Autodesk Fusion 360 part; units mm, degrees
(part 2 of 4)
  line L450 (2.2628, 34.1962) -> (6.5929, 31.6962)
  line L451 (6.5929, 31.6962) -> (10.923, 34.1962)
  line L452 (10.923, 34.1962) -> (10.923, 39.1962)
  line L453 (10.923, 39.1962) -> (6.5929, 41.6962)
  line L454 (17.2532, 41.6962) -> (12.923, 39.1962)
  line L455 (12.923, 39.1962) -> (12.923, 34.1962)
  line L456 (12.923, 34.1962) -> (17.2532, 31.6962)
  line L457 (17.2532, 31.6962) -> (21.5833, 34.1962)
  line L458 (21.5833, 34.1962) -> (21.5833, 39.1962)
  line L459 (21.5833, 39.1962) -> (17.2532, 41.6962)
  line L460 (27.9134, 41.6962) -> (23.5833, 39.1962)
  line L461 (23.5833, 39.1962) -> (23.5833, 34.1962)
  line L462 (23.5833, 34.1962) -> (27.9134, 31.6962)
  line L463 (27.9134, 31.6962) -> (32.2436, 34.1962)
  line L464 (32.2436, 34.1962) -> (32.2436, 39.1962)
  line L465 (32.2436, 39.1962) -> (27.9134, 41.6962)
  line L466 (38.5737, 41.6962) -> (34.2436, 39.1962)
  line L467 (34.2436, 39.1962) -> (34.2436, 34.1962)
  line L468 (34.2436, 34.1962) -> (38.5737, 31.6962)
  line L469 (38.5737, 31.6962) -> (42.9038, 34.1962)
  line L470 (42.9038, 34.1962) -> (42.9038, 39.1962)
  line L471 (42.9038, 39.1962) -> (38.5737, 41.6962)
  line L472 (49.2339, 41.6962) -> (44.9038, 39.1962)
  line L473 (44.9038, 39.1962) -> (44.9038, 34.1962)
  line L474 (44.9038, 34.1962) -> (49.2339, 31.6962)
  line L475 (49.2339, 31.6962) -> (53.5641, 34.1962)
  line L476 (53.5641, 34.1962) -> (53.5641, 39.1962)
  line L477 (53.5641, 39.1962) -> (49.2339, 41.6962)
  line L478 (59.8942, 41.6962) -> (55.5641, 39.1962)
  line L479 (55.5641, 39.1962) -> (55.5641, 34.1962)
  line L480 (55.5641, 34.1962) -> (59.8942, 31.6962)
  line L481 (59.8942, 31.6962) -> (64.2243, 34.1962)
  line L482 (64.2243, 34.1962) -> (64.2243, 39.1962)
  line L483 (64.2243, 39.1962) -> (59.8942, 41.6962)
  line L484 (70.5544, 41.6962) -> (66.2243, 39.1962)
  line L485 (66.2243, 39.1962) -> (66.2243, 34.1962)
  line L486 (66.2243, 34.1962) -> (70.5544, 31.6962)
  line L487 (70.5544, 31.6962) -> (74.8846, 34.1962)
  line L488 (74.8846, 34.1962) -> (74.8846, 39.1962)
  line L489 (74.8846, 39.1962) -> (70.5544, 41.6962)
  line L490 (81.2147, 41.6962) -> (76.8846, 39.1962)
  line L491 (76.8846, 39.1962) -> (76.8846, 34.1962)
  line L492 (76.8846, 34.1962) -> (81.2147, 31.6962)
  line L493 (81.2147, 31.6962) -> (85.5448, 34.1962)
  line L494 (85.5448, 34.1962) -> (85.5448, 39.1962)
  line L495 (85.5448, 39.1962) -> (81.2147, 41.6962)
  line L496 (91.875, 41.6962) -> (87.5448, 39.1962)
  line L497 (87.5448, 39.1962) -> (87.5448, 34.1962)
  line L498 (87.5448, 34.1962) -> (91.875, 31.6962)
  line L499 (91.875, 31.6962) -> (96.2051, 34.1962)
  line L500 (96.2051, 34.1962) -> (96.2051, 39.1962)
  line L501 (96.2051, 39.1962) -> (91.875, 41.6962)
  line L502 (102.5352, 41.6962) -> (98.2051, 39.1962)
  line L503 (98.2051, 39.1962) -> (98.2051, 34.1962)
  line L504 (98.2051, 34.1962) -> (102.5352, 31.6962)
  line L505 (102.5352, 31.6962) -> (106.8653, 34.1962)
  line L506 (106.8653, 34.1962) -> (106.8653, 39.1962)
  line L507 (106.8653, 39.1962) -> (102.5352, 41.6962)
  line L508 (-116, 50.9282) -> (-120.3301, 48.4282)
  line L509 (-120.3301, 48.4282) -> (-120.3301, 43.4282)
  line L510 (-120.3301, 43.4282) -> (-116, 40.9282)
  line L511 (-116, 40.9282) -> (-111.6699, 43.4282)
  line L512 (-111.6699, 43.4282) -> (-111.6699, 48.4282)
  line L513 (-111.6699, 48.4282) -> (-116, 50.9282)
  line L514 (-105.3397, 50.9282) -> (-109.6699, 48.4282)
  line L515 (-109.6699, 48.4282) -> (-109.6699, 43.4282)
  line L516 (-109.6699, 43.4282) -> (-105.3397, 40.9282)
  line L517 (-105.3397, 40.9282) -> (-101.0096, 43.4282)
  line L518 (-101.0096, 43.4282) -> (-101.0096, 48.4282)
  line L519 (-101.0096, 48.4282) -> (-105.3397, 50.9282)
  line L520 (-94.6795, 50.9282) -> (-99.0096, 48.4282)
  line L521 (-99.0096, 48.4282) -> (-99.0096, 43.4282)
  line L522 (-99.0096, 43.4282) -> (-94.6795, 40.9282)
  line L523 (-94.6795, 40.9282) -> (-90.3494, 43.4282)
  line L524 (-90.3494, 43.4282) -> (-90.3494, 48.4282)
  line L525 (-90.3494, 48.4282) -> (-94.6795, 50.9282)
  line L526 (-84.0192, 50.9282) -> (-88.3494, 48.4282)
  line L527 (-88.3494, 48.4282) -> (-88.3494, 43.4282)
  line L528 (-88.3494, 43.4282) -> (-84.0192, 40.9282)
  line L529 (-84.0192, 40.9282) -> (-79.6891, 43.4282)
  line L530 (-79.6891, 43.4282) -> (-79.6891, 48.4282)
  line L531 (-79.6891, 48.4282) -> (-84.0192, 50.9282)
  line L532 (-73.359, 50.9282) -> (-77.6891, 48.4282)
  line L533 (-77.6891, 48.4282) -> (-77.6891, 43.4282)
  line L534 (-77.6891, 43.4282) -> (-73.359, 40.9282)
  line L535 (-73.359, 40.9282) -> (-69.0289, 43.4282)
  line L536 (-69.0289, 43.4282) -> (-69.0289, 48.4282)
  line L537 (-69.0289, 48.4282) -> (-73.359, 50.9282)
  line L538 (-62.6987, 50.9282) -> (-67.0289, 48.4282)
  line L539 (-67.0289, 48.4282) -> (-67.0289, 43.4282)
  line L540 (-67.0289, 43.4282) -> (-62.6987, 40.9282)
  line L541 (-62.6987, 40.9282) -> (-58.3686, 43.4282)
  line L542 (-58.3686, 43.4282) -> (-58.3686, 48.4282)
  line L543 (-58.3686, 48.4282) -> (-62.6987, 50.9282)
  line L544 (-52.0385, 50.9282) -> (-56.3686, 48.4282)
  line L545 (-56.3686, 48.4282) -> (-56.3686, 43.4282)
  line L546 (-56.3686, 43.4282) -> (-52.0385, 40.9282)
  line L547 (-52.0385, 40.9282) -> (-47.7083, 43.4282)
  line L548 (-47.7083, 43.4282) -> (-47.7083, 48.4282)
  line L549 (-47.7083, 48.4282) -> (-52.0385, 50.9282)
  line L550 (-41.3782, 50.9282) -> (-45.7083, 48.4282)
  line L551 (-45.7083, 48.4282) -> (-45.7083, 43.4282)
  line L552 (-45.7083, 43.4282) -> (-41.3782, 40.9282)
  line L553 (-41.3782, 40.9282) -> (-37.0481, 43.4282)
  line L554 (-37.0481, 43.4282) -> (-37.0481, 48.4282)
  line L555 (-37.0481, 48.4282) -> (-41.3782, 50.9282)
  line L556 (-30.718, 50.9282) -> (-35.0481, 48.4282)
  line L557 (-35.0481, 48.4282) -> (-35.0481, 43.4282)
  line L558 (-35.0481, 43.4282) -> (-30.718, 40.9282)
  line L559 (-30.718, 40.9282) -> (-26.3878, 43.4282)
  line L560 (-26.3878, 43.4282) -> (-26.3878, 48.4282)
  line L561 (-26.3878, 48.4282) -> (-30.718, 50.9282)
  line L562 (-20.0577, 50.9282) -> (-24.3878, 48.4282)
  line L563 (-24.3878, 48.4282) -> (-24.3878, 43.4282)
  line L564 (-24.3878, 43.4282) -> (-20.0577, 40.9282)
  line L565 (-20.0577, 40.9282) -> (-15.7276, 43.4282)
  line L566 (-15.7276, 43.4282) -> (-15.7276, 48.4282)
  line L567 (-15.7276, 48.4282) -> (-20.0577, 50.9282)
  line L568 (-9.3975, 50.9282) -> (-13.7276, 48.4282)
  line L569 (-13.7276, 48.4282) -> (-13.7276, 43.4282)
  line L570 (-13.7276, 43.4282) -> (-9.3975, 40.9282)
  line L571 (-9.3975, 40.9282) -> (-5.0673, 43.4282)
  line L572 (-5.0673, 43.4282) -> (-5.0673, 48.4282)
  line L573 (-5.0673, 48.4282) -> (-9.3975, 50.9282)
  line L574 (1.2628, 50.9282) -> (-3.0673, 48.4282)
  line L575 (-3.0673, 48.4282) -> (-3.0673, 43.4282)
  line L576 (-3.0673, 43.4282) -> (1.2628, 40.9282)
  line L577 (1.2628, 40.9282) -> (5.5929, 43.4282)
  line L578 (5.5929, 43.4282) -> (5.5929, 48.4282)
  line L579 (5.5929, 48.4282) -> (1.2628, 50.9282)
  line L580 (11.923, 50.9282) -> (7.5929, 48.4282)
  line L581 (7.5929, 48.4282) -> (7.5929, 43.4282)
  line L582 (7.5929, 43.4282) -> (11.923, 40.9282)
  line L583 (11.923, 40.9282) -> (16.2532, 43.4282)
  line L584 (16.2532, 43.4282) -> (16.2532, 48.4282)
  line L585 (16.2532, 48.4282) -> (11.923, 50.9282)
  line L586 (22.5833, 50.9282) -> (18.2532, 48.4282)
  line L587 (18.2532, 48.4282) -> (18.2532, 43.4282)
  line L588 (18.2532, 43.4282) -> (22.5833, 40.9282)
  line L589 (22.5833, 40.9282) -> (26.9134, 43.4282)
  line L590 (26.9134, 43.4282) -> (26.9134, 48.4282)
  line L591 (26.9134, 48.4282) -> (22.5833, 50.9282)
  line L592 (33.2436, 50.9282) -> (28.9134, 48.4282)
  line L593 (28.9134, 48.4282) -> (28.9134, 43.4282)
  line L594 (28.9134, 43.4282) -> (33.2436, 40.9282)
  line L595 (33.2436, 40.9282) -> (37.5737, 43.4282)
  line L596 (37.5737, 43.4282) -> (37.5737, 48.4282)
  line L597 (37.5737, 48.4282) -> (33.2436, 50.9282)
  line L598 (43.9038, 50.9282) -> (39.5737, 48.4282)
  line L599 (39.5737, 48.4282) -> (39.5737, 43.4282)
  line L600 (39.5737, 43.4282) -> (43.9038, 40.9282)
  line L601 (43.9038, 40.9282) -> (48.2339, 43.4282)
  line L602 (48.2339, 43.4282) -> (48.2339, 48.4282)
  line L603 (48.2339, 48.4282) -> (43.9038, 50.9282)
  line L604 (54.5641, 50.9282) -> (50.2339, 48.4282)
  line L605 (50.2339, 48.4282) -> (50.2339, 43.4282)
  line L606 (50.2339, 43.4282) -> (54.5641, 40.9282)
  line L607 (54.5641, 40.9282) -> (58.8942, 43.4282)
  line L608 (58.8942, 43.4282) -> (58.8942, 48.4282)
  line L609 (58.8942, 48.4282) -> (54.5641, 50.9282)
  line L610 (65.2243, 50.9282) -> (60.8942, 48.4282)
  line L611 (60.8942, 48.4282) -> (60.8942, 43.4282)
  line L612 (60.8942, 43.4282) -> (65.2243, 40.9282)
  line L613 (65.2243, 40.9282) -> (69.5544, 43.4282)
  line L614 (69.5544, 43.4282) -> (69.5544, 48.4282)
  line L615 (69.5544, 48.4282) -> (65.2243, 50.9282)
  line L616 (75.8846, 50.9282) -> (71.5544, 48.4282)
  line L617 (71.5544, 48.4282) -> (71.5544, 43.4282)
  line L618 (71.5544, 43.4282) -> (75.8846, 40.9282)
  line L619 (75.8846, 40.9282) -> (80.2147, 43.4282)
  line L620 (80.2147, 43.4282) -> (80.2147, 48.4282)
  line L621 (80.2147, 48.4282) -> (75.8846, 50.9282)
  line L622 (86.5448, 50.9282) -> (82.2147, 48.4282)
  line L623 (82.2147, 48.4282) -> (82.2147, 43.4282)
  line L624 (82.2147, 43.4282) -> (86.5448, 40.9282)
  line L625 (86.5448, 40.9282) -> (90.875, 43.4282)
  line L626 (90.875, 43.4282) -> (90.875, 48.4282)
  line L627 (90.875, 48.4282) -> (86.5448, 50.9282)
  line L628 (97.2051, 50.9282) -> (92.875, 48.4282)
  line L629 (92.875, 48.4282) -> (92.875, 43.4282)
  line L630 (92.875, 43.4282) -> (97.2051, 40.9282)
  line L631 (97.2051, 40.9282) -> (101.5352, 43.4282)
  line L632 (101.5352, 43.4282) -> (101.5352, 48.4282)
  line L633 (101.5352, 48.4282) -> (97.2051, 50.9282)
  line L634 (-110.6699, 60.1603) -> (-115, 57.6603)
  line L635 (-115, 57.6603) -> (-115, 52.6603)
  line L636 (-115, 52.6603) -> (-110.6699, 50.1603)
  line L637 (-110.6699, 50.1603) -> (-106.3397, 52.6603)
  line L638 (-106.3397, 52.6603) -> (-106.3397, 57.6603)
  line L639 (-106.3397, 57.6603) -> (-110.6699, 60.1603)
  line L640 (-100.0096, 60.1603) -> (-104.3397, 57.6603)
  line L641 (-104.3397, 57.6603) -> (-104.3397, 52.6603)
  line L642 (-104.3397, 52.6603) -> (-100.0096, 50.1603)
  line L643 (-100.0096, 50.1603) -> (-95.6795, 52.6603)
  line L644 (-95.6795, 52.6603) -> (-95.6795, 57.6603)
  line L645 (-95.6795, 57.6603) -> (-100.0096, 60.1603)
  line L646 (-89.3494, 60.1603) -> (-93.6795, 57.6603)
  line L647 (-93.6795, 57.6603) -> (-93.6795, 52.6603)
  line L648 (-93.6795, 52.6603) -> (-89.3494, 50.1603)
  line L649 (-89.3494, 50.1603) -> (-85.0192, 52.6603)
  line L650 (-85.0192, 52.6603) -> (-85.0192, 57.6603)
  line L651 (-85.0192, 57.6603) -> (-89.3494, 60.1603)
  line L652 (-78.6891, 60.1603) -> (-83.0192, 57.6603)
  line L653 (-83.0192, 57.6603) -> (-83.0192, 52.6603)
  line L654 (-83.0192, 52.6603) -> (-78.6891, 50.1603)
  line L655 (-78.6891, 50.1603) -> (-74.359, 52.6603)
  line L656 (-74.359, 52.6603) -> (-74.359, 57.6603)
  line L657 (-74.359, 57.6603) -> (-78.6891, 60.1603)
  line L658 (-68.0289, 60.1603) -> (-72.359, 57.6603)
  line L659 (-72.359, 57.6603) -> (-72.359, 52.6603)
  line L660 (-72.359, 52.6603) -> (-68.0289, 50.1603)
  line L661 (-68.0289, 50.1603) -> (-63.6987, 52.6603)
  line L662 (-63.6987, 52.6603) -> (-63.6987, 57.6603)
  line L663 (-63.6987, 57.6603) -> (-68.0289, 60.1603)
  line L664 (-57.3686, 60.1603) -> (-61.6987, 57.6603)
  line L665 (-61.6987, 57.6603) -> (-61.6987, 52.6603)
  line L666 (-61.6987, 52.6603) -> (-57.3686, 50.1603)
  line L667 (-57.3686, 50.1603) -> (-53.0385, 52.6603)
  line L668 (-53.0385, 52.6603) -> (-53.0385, 57.6603)
  line L669 (-53.0385, 57.6603) -> (-57.3686, 60.1603)
  line L670 (-46.7083, 60.1603) -> (-51.0385, 57.6603)
  line L671 (-51.0385, 57.6603) -> (-51.0385, 52.6603)
  line L672 (-51.0385, 52.6603) -> (-46.7083, 50.1603)
  line L673 (-46.7083, 50.1603) -> (-42.3782, 52.6603)
  line L674 (-42.3782, 52.6603) -> (-42.3782, 57.6603)
  line L675 (-42.3782, 57.6603) -> (-46.7083, 60.1603)
  line L676 (-36.0481, 60.1603) -> (-40.3782, 57.6603)
  line L677 (-40.3782, 57.6603) -> (-40.3782, 52.6603)
  line L678 (-40.3782, 52.6603) -> (-36.0481, 50.1603)
  line L679 (-36.0481, 50.1603) -> (-31.718, 52.6603)
  line L680 (-31.718, 52.6603) -> (-31.718, 57.6603)
  line L681 (-31.718, 57.6603) -> (-36.0481, 60.1603)
  line L682 (-25.3878, 60.1603) -> (-29.718, 57.6603)
  line L683 (-29.718, 57.6603) -> (-29.718, 52.6603)
  line L684 (-29.718, 52.6603) -> (-25.3878, 50.1603)
  line L685 (-25.3878, 50.1603) -> (-21.0577, 52.6603)
  line L686 (-21.0577, 52.6603) -> (-21.0577, 57.6603)
  line L687 (-21.0577, 57.6603) -> (-25.3878, 60.1603)
  line L688 (-14.7276, 60.1603) -> (-19.0577, 57.6603)
  line L689 (-19.0577, 57.6603) -> (-19.0577, 52.6603)
  line L690 (-19.0577, 52.6603) -> (-14.7276, 50.1603)
  line L691 (-14.7276, 50.1603) -> (-10.3975, 52.6603)
  line L692 (-10.3975, 52.6603) -> (-10.3975, 57.6603)
  line L693 (-10.3975, 57.6603) -> (-14.7276, 60.1603)
  line L694 (-4.0673, 60.1603) -> (-8.3975, 57.6603)
  line L695 (-8.3975, 57.6603) -> (-8.3975, 52.6603)
  line L696 (-8.3975, 52.6603) -> (-4.0673, 50.1603)
  line L697 (-4.0673, 50.1603) -> (0.2628, 52.6603)
  line L698 (0.2628, 52.6603) -> (0.2628, 57.6603)
  line L699 (0.2628, 57.6603) -> (-4.0673, 60.1603)
  line L700 (6.5929, 60.1603) -> (2.2628, 57.6603)
  line L701 (2.2628, 57.6603) -> (2.2628, 52.6603)
  line L702 (2.2628, 52.6603) -> (6.5929, 50.1603)
  line L703 (6.5929, 50.1603) -> (10.923, 52.6603)
  line L704 (10.923, 52.6603) -> (10.923, 57.6603)
  line L705 (10.923, 57.6603) -> (6.5929, 60.1603)
  line L706 (17.2532, 60.1603) -> (12.923, 57.6603)
  line L707 (12.923, 57.6603) -> (12.923, 52.6603)
  line L708 (12.923, 52.6603) -> (17.2532, 50.1603)
  line L709 (17.2532, 50.1603) -> (21.5833, 52.6603)
  line L710 (21.5833, 52.6603) -> (21.5833, 57.6603)
  line L711 (21.5833, 57.6603) -> (17.2532, 60.1603)
  line L712 (27.9134, 60.1603) -> (23.5833, 57.6603)
  line L713 (23.5833, 57.6603) -> (23.5833, 52.6603)
  line L714 (23.5833, 52.6603) -> (27.9134, 50.1603)
  line L715 (27.9134, 50.1603) -> (32.2436, 52.6603)
  line L716 (32.2436, 52.6603) -> (32.2436, 57.6603)
  line L717 (32.2436, 57.6603) -> (27.9134, 60.1603)
  line L718 (38.5737, 60.1603) -> (34.2436, 57.6603)
  line L719 (34.2436, 57.6603) -> (34.2436, 52.6603)
  line L720 (34.2436, 52.6603) -> (38.5737, 50.1603)
  line L721 (38.5737, 50.1603) -> (42.9038, 52.6603)
  line L722 (42.9038, 52.6603) -> (42.9038, 57.6603)
  line L723 (42.9038, 57.6603) -> (38.5737, 60.1603)
  line L724 (49.2339, 60.1603) -> (44.9038, 57.6603)
  line L725 (44.9038, 57.6603) -> (44.9038, 52.6603)
  line L726 (44.9038, 52.6603) -> (49.2339, 50.1603)
  line L727 (49.2339, 50.1603) -> (53.5641, 52.6603)
  line L728 (53.5641, 52.6603) -> (53.5641, 57.6603)
  line L729 (53.5641, 57.6603) -> (49.2339, 60.1603)
  line L730 (59.8942, 60.1603) -> (55.5641, 57.6603)
  line L731 (55.5641, 57.6603) -> (55.5641, 52.6603)
  line L732 (55.5641, 52.6603) -> (59.8942, 50.1603)
  line L733 (59.8942, 50.1603) -> (64.2243, 52.6603)
  line L734 (64.2243, 52.6603) -> (64.2243, 57.6603)
  line L735 (64.2243, 57.6603) -> (59.8942, 60.1603)
  line L736 (70.5544, 60.1603) -> (66.2243, 57.6603)
  line L737 (66.2243, 57.6603) -> (66.2243, 52.6603)
  line L738 (66.2243, 52.6603) -> (70.5544, 50.1603)
  line L739 (70.5544, 50.1603) -> (74.8846, 52.6603)
  line L740 (74.8846, 52.6603) -> (74.8846, 57.6603)
  line L741 (74.8846, 57.6603) -> (70.5544, 60.1603)
  line L742 (81.2147, 60.1603) -> (76.8846, 57.6603)
  line L743 (76.8846, 57.6603) -> (76.8846, 52.6603)
  line L744 (76.8846, 52.6603) -> (81.2147, 50.1603)
  line L745 (81.2147, 50.1603) -> (85.5448, 52.6603)
  line L746 (85.5448, 52.6603) -> (85.5448, 57.6603)
  line L747 (85.5448, 57.6603) -> (81.2147, 60.1603)
  line L748 (91.875, 60.1603) -> (87.5448, 57.6603)
  line L749 (87.5448, 57.6603) -> (87.5448, 52.6603)
  line L750 (87.5448, 52.6603) -> (91.875, 50.1603)
  line L751 (91.875, 50.1603) -> (96.2051, 52.6603)
  line L752 (96.2051, 52.6603) -> (96.2051, 57.6603)
  line L753 (96.2051, 57.6603) -> (91.875, 60.1603)
  line L754 (102.5352, 60.1603) -> (98.2051, 57.6603)
  line L755 (98.2051, 57.6603) -> (98.2051, 52.6603)
  line L756 (98.2051, 52.6603) -> (102.5352, 50.1603)
  line L757 (102.5352, 50.1603) -> (106.8653, 52.6603)
  line L758 (106.8653, 52.6603) -> (106.8653, 57.6603)
  line L759 (106.8653, 57.6603) -> (102.5352, 60.1603)
  line L760 (-116, 69.3923) -> (-120.3301, 66.8923)
  line L761 (-120.3301, 66.8923) -> (-120.3301, 61.8923)
  line L762 (-120.3301, 61.8923) -> (-116, 59.3923)
  line L763 (-116, 59.3923) -> (-111.6699, 61.8923)
  line L764 (-111.6699, 61.8923) -> (-111.6699, 66.8923)
  line L765 (-111.6699, 66.8923) -> (-116, 69.3923)
  line L766 (-105.3397, 69.3923) -> (-109.6699, 66.8923)
  line L767 (-109.6699, 66.8923) -> (-109.6699, 61.8923)
  line L768 (-109.6699, 61.8923) -> (-105.3397, 59.3923)
  line L769 (-105.3397, 59.3923) -> (-101.0096, 61.8923)
  line L770 (-101.0096, 61.8923) -> (-101.0096, 66.8923)
  line L771 (-101.0096, 66.8923) -> (-105.3397, 69.3923)
  line L772 (-94.6795, 69.3923) -> (-99.0096, 66.8923)
  line L773 (-99.0096, 66.8923) -> (-99.0096, 61.8923)
  line L774 (-99.0096, 61.8923) -> (-94.6795, 59.3923)
  line L775 (-94.6795, 59.3923) -> (-90.3494, 61.8923)
  line L776 (-90.3494, 61.8923) -> (-90.3494, 66.8923)
  line L777 (-90.3494, 66.8923) -> (-94.6795, 69.3923)
  line L778 (-84.0192, 69.3923) -> (-88.3494, 66.8923)
  line L779 (-88.3494, 66.8923) -> (-88.3494, 61.8923)
  line L780 (-88.3494, 61.8923) -> (-84.0192, 59.3923)
  line L781 (-84.0192, 59.3923) -> (-79.6891, 61.8923)
  line L782 (-79.6891, 61.8923) -> (-79.6891, 66.8923)
  line L783 (-79.6891, 66.8923) -> (-84.0192, 69.3923)
  line L784 (-73.359, 69.3923) -> (-77.6891, 66.8923)
  line L785 (-77.6891, 66.8923) -> (-77.6891, 61.8923)
  line L786 (-77.6891, 61.8923) -> (-73.359, 59.3923)
  line L787 (-73.359, 59.3923) -> (-69.0289, 61.8923)
  line L788 (-69.0289, 61.8923) -> (-69.0289, 66.8923)
  line L789 (-69.0289, 66.8923) -> (-73.359, 69.3923)
  line L790 (-62.6987, 69.3923) -> (-67.0289, 66.8923)
  line L791 (-67.0289, 66.8923) -> (-67.0289, 61.8923)
  line L792 (-67.0289, 61.8923) -> (-62.6987, 59.3923)
  line L793 (-62.6987, 59.3923) -> (-58.3686, 61.8923)
  line L794 (-58.3686, 61.8923) -> (-58.3686, 66.8923)
  line L795 (-58.3686, 66.8923) -> (-62.6987, 69.3923)
  line L796 (-52.0385, 69.3923) -> (-56.3686, 66.8923)
  line L797 (-56.3686, 66.8923) -> (-56.3686, 61.8923)
  line L798 (-56.3686, 61.8923) -> (-52.0385, 59.3923)
  line L799 (-52.0385, 59.3923) -> (-47.7083, 61.8923)
  line L800 (-47.7083, 61.8923) -> (-47.7083, 66.8923)
  line L801 (-47.7083, 66.8923) -> (-52.0385, 69.3923)
  line L802 (-41.3782, 69.3923) -> (-45.7083, 66.8923)
  line L803 (-45.7083, 66.8923) -> (-45.7083, 61.8923)
  line L804 (-45.7083, 61.8923) -> (-41.3782, 59.3923)
  line L805 (-41.3782, 59.3923) -> (-37.0481, 61.8923)
  line L806 (-37.0481, 61.8923) -> (-37.0481, 66.8923)
  line L807 (-37.0481, 66.8923) -> (-41.3782, 69.3923)
  line L808 (-30.718, 69.3923) -> (-35.0481, 66.8923)
  line L809 (-35.0481, 66.8923) -> (-35.0481, 61.8923)
  line L810 (-35.0481, 61.8923) -> (-30.718, 59.3923)
  line L811 (-30.718, 59.3923) -> (-26.3878, 61.8923)
  line L812 (-26.3878, 61.8923) -> (-26.3878, 66.8923)
  line L813 (-26.3878, 66.8923) -> (-30.718, 69.3923)
  line L814 (-20.0577, 69.3923) -> (-24.3878, 66.8923)
  line L815 (-24.3878, 66.8923) -> (-24.3878, 61.8923)
  line L816 (-24.3878, 61.8923) -> (-20.0577, 59.3923)
  line L817 (-20.0577, 59.3923) -> (-15.7276, 61.8923)
  line L818 (-15.7276, 61.8923) -> (-15.7276, 66.8923)
  line L819 (-15.7276, 66.8923) -> (-20.0577, 69.3923)
  line L820 (-9.3975, 69.3923) -> (-13.7276, 66.8923)
  line L821 (-13.7276, 66.8923) -> (-13.7276, 61.8923)
  line L822 (-13.7276, 61.8923) -> (-9.3975, 59.3923)
  line L823 (-9.3975, 59.3923) -> (-5.0673, 61.8923)
  line L824 (-5.0673, 61.8923) -> (-5.0673, 66.8923)
  line L825 (-5.0673, 66.8923) -> (-9.3975, 69.3923)
  line L826 (1.2628, 69.3923) -> (-3.0673, 66.8923)
  line L827 (-3.0673, 66.8923) -> (-3.0673, 61.8923)
  line L828 (-3.0673, 61.8923) -> (1.2628, 59.3923)
  line L829 (1.2628, 59.3923) -> (5.5929, 61.8923)
  line L830 (5.5929, 61.8923) -> (5.5929, 66.8923)
  line L831 (5.5929, 66.8923) -> (1.2628, 69.3923)
  line L832 (11.923, 69.3923) -> (7.5929, 66.8923)
  line L833 (7.5929, 66.8923) -> (7.5929, 61.8923)
  line L834 (7.5929, 61.8923) -> (11.923, 59.3923)
  line L835 (11.923, 59.3923) -> (16.2532, 61.8923)
  line L836 (16.2532, 61.8923) -> (16.2532, 66.8923)
  line L837 (16.2532, 66.8923) -> (11.923, 69.3923)
  line L838 (22.5833, 69.3923) -> (18.2532, 66.8923)
  line L839 (18.2532, 66.8923) -> (18.2532, 61.8923)
  line L840 (18.2532, 61.8923) -> (22.5833, 59.3923)
  line L841 (22.5833, 59.3923) -> (26.9134, 61.8923)
  line L842 (26.9134, 61.8923) -> (26.9134, 66.8923)
  line L843 (26.9134, 66.8923) -> (22.5833, 69.3923)
  line L844 (33.2436, 69.3923) -> (28.9134, 66.8923)
  line L845 (28.9134, 66.8923) -> (28.9134, 61.8923)
  line L846 (28.9134, 61.8923) -> (33.2436, 59.3923)
  line L847 (33.2436, 59.3923) -> (37.5737, 61.8923)
  line L848 (37.5737, 61.8923) -> (37.5737, 66.8923)
  line L849 (37.5737, 66.8923) -> (33.2436, 69.3923)
  line L850 (43.9038, 69.3923) -> (39.5737, 66.8923)
  line L851 (39.5737, 66.8923) -> (39.5737, 61.8923)
  line L852 (39.5737, 61.8923) -> (43.9038, 59.3923)
  line L853 (43.9038, 59.3923) -> (48.2339, 61.8923)
  line L854 (48.2339, 61.8923) -> (48.2339, 66.8923)
  line L855 (48.2339, 66.8923) -> (43.9038, 69.3923)
  line L856 (54.5641, 69.3923) -> (50.2339, 66.8923)
  line L857 (50.2339, 66.8923) -> (50.2339, 61.8923)
  line L858 (50.2339, 61.8923) -> (54.5641, 59.3923)
  line L859 (54.5641, 59.3923) -> (58.8942, 61.8923)
  line L860 (58.8942, 61.8923) -> (58.8942, 66.8923)
  line L861 (58.8942, 66.8923) -> (54.5641, 69.3923)
  line L862 (65.2243, 69.3923) -> (60.8942, 66.8923)
  line L863 (60.8942, 66.8923) -> (60.8942, 61.8923)
  line L864 (60.8942, 61.8923) -> (65.2243, 59.3923)
  line L865 (65.2243, 59.3923) -> (69.5544, 61.8923)
  line L866 (69.5544, 61.8923) -> (69.5544, 66.8923)
  line L867 (69.5544, 66.8923) -> (65.2243, 69.3923)
  line L868 (75.8846, 69.3923) -> (71.5544, 66.8923)
  line L869 (71.5544, 66.8923) -> (71.5544, 61.8923)
  line L870 (71.5544, 61.8923) -> (75.8846, 59.3923)
  line L871 (75.8846, 59.3923) -> (80.2147, 61.8923)
  line L872 (80.2147, 61.8923) -> (80.2147, 66.8923)
  line L873 (80.2147, 66.8923) -> (75.8846, 69.3923)
  line L874 (86.5448, 69.3923) -> (82.2147, 66.8923)
  line L875 (82.2147, 66.8923) -> (82.2147, 61.8923)
  line L876 (82.2147, 61.8923) -> (86.5448, 59.3923)
  line L877 (86.5448, 59.3923) -> (90.875, 61.8923)
  line L878 (90.875, 61.8923) -> (90.875, 66.8923)
  line L879 (90.875, 66.8923) -> (86.5448, 69.3923)
  line L880 (97.2051, 69.3923) -> (92.875, 66.8923)
  line L881 (92.875, 66.8923) -> (92.875, 61.8923)
  line L882 (92.875, 61.8923) -> (97.2051, 59.3923)
  line L883 (97.2051, 59.3923) -> (101.5352, 61.8923)
  line L884 (101.5352, 61.8923) -> (101.5352, 66.8923)
  line L885 (101.5352, 66.8923) -> (97.2051, 69.3923)
  line L886 (-110.6699, 78.6244) -> (-115, 76.1244)
  line L887 (-115, 76.1244) -> (-115, 71.1244)
  line L888 (-115, 71.1244) -> (-110.6699, 68.6244)
  line L889 (-110.6699, 68.6244) -> (-106.3397, 71.1244)
  line L890 (-106.3397, 71.1244) -> (-106.3397, 76.1244)
  line L891 (-106.3397, 76.1244) -> (-110.6699, 78.6244)
  line L892 (-100.0096, 78.6244) -> (-104.3397, 76.1244)
  line L893 (-104.3397, 76.1244) -> (-104.3397, 71.1244)
  line L894 (-104.3397, 71.1244) -> (-100.0096, 68.6244)
  line L895 (-100.0096, 68.6244) -> (-95.6795, 71.1244)
  line L896 (-95.6795, 71.1244) -> (-95.6795, 76.1244)
  line L897 (-95.6795, 76.1244) -> (-100.0096, 78.6244)
  line L898 (-89.3494, 78.6244) -> (-93.6795, 76.1244)
  line L899 (-93.6795, 76.1244) -> (-93.6795, 71.1244)
  line L900 (-93.6795, 71.1244) -> (-89.3494, 68.6244)
  line L901 (-89.3494, 68.6244) -> (-85.0192, 71.1244)
  line L902 (-85.0192, 71.1244) -> (-85.0192, 76.1244)
  line L903 (-85.0192, 76.1244) -> (-89.3494, 78.6244)
  line L904 (-78.6891, 78.6244) -> (-83.0192, 76.1244)
  line L905 (-83.0192, 76.1244) -> (-83.0192, 71.1244)
  line L906 (-83.0192, 71.1244) -> (-78.6891, 68.6244)
  line L907 (-78.6891, 68.6244) -> (-74.359, 71.1244)
  line L908 (-74.359, 71.1244) -> (-74.359, 76.1244)
  line L909 (-74.359, 76.1244) -> (-78.6891, 78.6244)
  line L910 (-68.0289, 78.6244) -> (-72.359, 76.1244)
  line L911 (-72.359, 76.1244) -> (-72.359, 71.1244)
  line L912 (-72.359, 71.1244) -> (-68.0289, 68.6244)
  line L913 (-68.0289, 68.6244) -> (-63.6987, 71.1244)
  line L914 (-63.6987, 71.1244) -> (-63.6987, 76.1244)
  line L915 (-63.6987, 76.1244) -> (-68.0289, 78.6244)
  line L916 (-57.3686, 78.6244) -> (-61.6987, 76.1244)
  line L917 (-61.6987, 76.1244) -> (-61.6987, 71.1244)
  line L918 (-61.6987, 71.1244) -> (-57.3686, 68.6244)
  line L919 (-57.3686, 68.6244) -> (-53.0385, 71.1244)
  line L920 (-53.0385, 71.1244) -> (-53.0385, 76.1244)
  line L921 (-53.0385, 76.1244) -> (-57.3686, 78.6244)
  line L922 (-46.7083, 78.6244) -> (-51.0385, 76.1244)
  line L923 (-51.0385, 76.1244) -> (-51.0385, 71.1244)
  line L924 (-51.0385, 71.1244) -> (-46.7083, 68.6244)
  line L925 (-46.7083, 68.6244) -> (-42.3782, 71.1244)
  line L926 (-42.3782, 71.1244) -> (-42.3782, 76.1244)
  line L927 (-42.3782, 76.1244) -> (-46.7083, 78.6244)
  line L928 (-36.0481, 78.6244) -> (-40.3782, 76.1244)
  line L929 (-40.3782, 76.1244) -> (-40.3782, 71.1244)
  line L930 (-40.3782, 71.1244) -> (-36.0481, 68.6244)
  line L931 (-36.0481, 68.6244) -> (-31.718, 71.1244)
  line L932 (-31.718, 71.1244) -> (-31.718, 76.1244)
  line L933 (-31.718, 76.1244) -> (-36.0481, 78.6244)
  line L934 (-25.3878, 78.6244) -> (-29.718, 76.1244)
  line L935 (-29.718, 76.1244) -> (-29.718, 71.1244)
  line L936 (-29.718, 71.1244) -> (-25.3878, 68.6244)
  line L937 (-25.3878, 68.6244) -> (-21.0577, 71.1244)
  line L938 (-21.0577, 71.1244) -> (-21.0577, 76.1244)
  line L939 (-21.0577, 76.1244) -> (-25.3878, 78.6244)
  line L940 (-14.7276, 78.6244) -> (-19.0577, 76.1244)
  line L941 (-19.0577, 76.1244) -> (-19.0577, 71.1244)
  line L942 (-19.0577, 71.1244) -> (-14.7276, 68.6244)
  line L943 (-14.7276, 68.6244) -> (-10.3975, 71.1244)
  line L944 (-10.3975, 71.1244) -> (-10.3975, 76.1244)
  line L945 (-10.3975, 76.1244) -> (-14.7276, 78.6244)
  line L946 (-4.0673, 78.6244) -> (-8.3975, 76.1244)
  line L947 (-8.3975, 76.1244) -> (-8.3975, 71.1244)
  line L948 (-8.3975, 71.1244) -> (-4.0673, 68.6244)
  line L949 (-4.0673, 68.6244) -> (0.2628, 71.1244)
  line L950 (0.2628, 71.1244) -> (0.2628, 76.1244)
  line L951 (0.2628, 76.1244) -> (-4.0673, 78.6244)
  line L952 (6.5929, 78.6244) -> (2.2628, 76.1244)
  line L953 (2.2628, 76.1244) -> (2.2628, 71.1244)
  line L954 (2.2628, 71.1244) -> (6.5929, 68.6244)
  line L955 (6.5929, 68.6244) -> (10.923, 71.1244)
  line L956 (10.923, 71.1244) -> (10.923, 76.1244)
  line L957 (10.923, 76.1244) -> (6.5929, 78.6244)
  line L958 (17.2532, 78.6244) -> (12.923, 76.1244)
  line L959 (12.923, 76.1244) -> (12.923, 71.1244)
  line L960 (12.923, 71.1244) -> (17.2532, 68.6244)
  line L961 (17.2532, 68.6244) -> (21.5833, 71.1244)
  line L962 (21.5833, 71.1244) -> (21.5833, 76.1244)
  line L963 (21.5833, 76.1244) -> (17.2532, 78.6244)
  line L964 (27.9134, 78.6244) -> (23.5833, 76.1244)
  line L965 (23.5833, 76.1244) -> (23.5833, 71.1244)
  line L966 (23.5833, 71.1244) -> (27.9134, 68.6244)
  line L967 (27.9134, 68.6244) -> (32.2436, 71.1244)
  line L968 (32.2436, 71.1244) -> (32.2436, 76.1244)
  line L969 (32.2436, 76.1244) -> (27.9134, 78.6244)
  line L970 (38.5737, 78.6244) -> (34.2436, 76.1244)
  line L971 (34.2436, 76.1244) -> (34.2436, 71.1244)
  line L972 (34.2436, 71.1244) -> (38.5737, 68.6244)
  line L973 (38.5737, 68.6244) -> (42.9038, 71.1244)
  line L974 (42.9038, 71.1244) -> (42.9038, 76.1244)
  line L975 (42.9038, 76.1244) -> (38.5737, 78.6244)
  line L976 (49.2339, 78.6244) -> (44.9038, 76.1244)
  line L977 (44.9038, 76.1244) -> (44.9038, 71.1244)
  line L978 (44.9038, 71.1244) -> (49.2339, 68.6244)
  line L979 (49.2339, 68.6244) -> (53.5641, 71.1244)
  line L980 (53.5641, 71.1244) -> (53.5641, 76.1244)
  line L981 (53.5641, 76.1244) -> (49.2339, 78.6244)
  line L982 (59.8942, 78.6244) -> (55.5641, 76.1244)
  line L983 (55.5641, 76.1244) -> (55.5641, 71.1244)
  line L984 (55.5641, 71.1244) -> (59.8942, 68.6244)
  line L985 (59.8942, 68.6244) -> (64.2243, 71.1244)
  line L986 (64.2243, 71.1244) -> (64.2243, 76.1244)
  line L987 (64.2243, 76.1244) -> (59.8942, 78.6244)
  line L988 (70.5544, 78.6244) -> (66.2243, 76.1244)
  line L989 (66.2243, 76.1244) -> (66.2243, 71.1244)
  line L990 (66.2243, 71.1244) -> (70.5544, 68.6244)
  line L991 (70.5544, 68.6244) -> (74.8846, 71.1244)
  line L992 (74.8846, 71.1244) -> (74.8846, 76.1244)
  line L993 (74.8846, 76.1244) -> (70.5544, 78.6244)
  line L994 (81.2147, 78.6244) -> (76.8846, 76.1244)
  line L995 (76.8846, 76.1244) -> (76.8846, 71.1244)
  line L996 (76.8846, 71.1244) -> (81.2147, 68.6244)
  line L997 (81.2147, 68.6244) -> (85.5448, 71.1244)
  line L998 (85.5448, 71.1244) -> (85.5448, 76.1244)
  line L999 (85.5448, 76.1244) -> (81.2147, 78.6244)
  line L1000 (91.875, 78.6244) -> (87.5448, 76.1244)
  line L1001 (87.5448, 76.1244) -> (87.5448, 71.1244)
  line L1002 (87.5448, 71.1244) -> (91.875, 68.6244)
  line L1003 (91.875, 68.6244) -> (96.2051, 71.1244)
  line L1004 (96.2051, 71.1244) -> (96.2051, 76.1244)
  line L1005 (96.2051, 76.1244) -> (91.875, 78.6244)
  line L1006 (102.5352, 78.6244) -> (98.2051, 76.1244)
  line L1007 (98.2051, 76.1244) -> (98.2051, 71.1244)
  line L1008 (98.2051, 71.1244) -> (102.5352, 68.6244)
  line L1009 (102.5352, 68.6244) -> (106.8653, 71.1244)
  line L1010 (106.8653, 71.1244) -> (106.8653, 76.1244)
  line L1011 (106.8653, 76.1244) -> (102.5352, 78.6244)
extrude "拉伸30" cut sketch "草图30" against normal blind 3 contours L4 L5 L6 L7 L8 L9 | L10 L11 L12 L13 L14 L15 | L16 L17 L18 L19 L20 L21 | L22 L23 L24 L25 L26 L27 | L28 L29 L30 L31 L32 L33 | L34 L35 L36 L37 L38 L39 | L40 L41 L42 L43 L44 L45 | L46 L47 L48 L49 L50 L51 | L52 L53 L54 L55 L56 L57 | L58 L59 L60 L61 L62 L63 | L64 L65 L66 L67 L68 L69 | L70 L71 L72 L73 L74 L75 | L76 L77 L78 L79 L80 L81 | L82 L83 L84 L85 L86 L87 | L88 L89 L90 L91 L92 L93 | L94 L95 L96 L97 L98 L99 | L100 L101 L102 L103 L104 L105 | L106 L107 L108 L109 L110 L111 | L112 L113 L114 L115 L116 L117 | L118 L119 L120 L121 L122 L123 | L124 L125 L126 L127 L128 L129 | L130 L131 L132 L133 L134 L135 | L136 L137 L138 L139 L140 L141 | L142 L143 L144 L145 L146 L147 | L148 L149 L150 L151 L152 L153 | L154 L155 L156 L157 L158 L159 | L160 L161 L162 L163 L164 L165 | L166 L167 L168 L169 L170 L171 | L172 L173 L174 L175 L176 L177 | L178 L179 L180 L181 L182 L183 | L184 L185 L186 L187 L188 L189 | L190 L191 L192 L193 L194 L195 | L196 L197 L198 L199 L200 L201 | L202 L203 L204 L205 L206 L207 | L208 L209 L210 L211 L212 L213 | L214 L215 L216 L217 L218 L219 | L220 L221 L222 L223 L224 L225 | L226 L227 L228 L229 L230 L231 | L232 L233 L234 L235 L236 L237 | L238 L239 L240 L241 L242 L243 | L244 L245 L246 L247 L248 L249 | L250 L251 L252 L253 L254 L255 | L256 L257 L258 L259 L260 L261 | L262 L263 L264 L265 L266 L267 | L268 L269 L270 L271 L272 L273 | L274 L275 L276 L277 L278 L279 | L280 L281 L282 L283 L284 L285 | L286 L287 L288 L289 L290 L291 | L292 L293 L294 L295 L296 L297 | L298 L299 L300 L301 L302 L303 | L304 L305 L306 L307 L308 L309 | L310 L311 L312 L313 L314 L315 | L316 L317 L318 L319 L320 L321 | L322 L323 L324 L325 L326 L327 | L328 L329 L330 L331 L332 L333 | L334 L335 L336 L337 L338 L339 | L340 L341 L342 L343 L344 L345 | L346 L347 L348 L349 L350 L351 | L352 L353 L354 L355 L356 L357 | L358 L359 L360 L361 L362 L363 | L364 L365 L366 L367 L368 L369 | L370 L371 L372 L373 L374 L375 | L376 L377 L378 L379 L380 L381 | L382 L383 L384 L385 L386 L387 | L388 L389 L390 L391 L392 L393 | L394 L395 L396 L397 L398 L399 | L400 L401 L402 L403 L404 L405 | L406 L407 L408 L409 L410 L411 | L412 L413 L414 L415 L416 L417 | L418 L419 L420 L421 L422 L423 | L424 L425 L426 L427 L428 L429 | L430 L431 L432 L433 L434 L435 | L436 L437 L438 L439 L440 L441 | L442 L443 L444 L445 L446 L447 | L448 L449 L450 L451 L452 L453 | L454 L455 L456 L457 L458 L459 | L460 L461 L462 L463 L464 L465 | L466 L467 L468 L469 L470 L471 | L472 L473 L474 L475 L476 L477 | L478 L479 L480 L481 L482 L483 | L484 L485 L486 L487 L488 L489 | L490 L491 L492 L493 L494 L495 | L496 L497 L498 L499 L500 L501 | L502 L503 L504 L505 L506 L507 | L508 L509 L510 L511 L512 L513 | L514 L515 L516 L517 L518 L519 | L520 L521 L522 L523 L524 L525 | L526 L527 L528 L529 L530 L531 | L532 L533 L534 L535 L536 L537 | L538 L539 L540 L541 L542 L543 | L544 L545 L546 L547 L548 L549 | L550 L551 L552 L553 L554 L555 | L556 L557 L558 L559 L560 L561 | L562 L563 L564 L565 L566 L567 | L568 L569 L570 L571 L572 L573 | L574 L575 L576 L577 L578 L579 | L580 L581 L582 L583 L584 L585 | L586 L587 L588 L589 L590 L591 | L592 L593 L594 L595 L596 L597 | L598 L599 L600 L601 L602 L603 | L604 L605 L606 L607 L608 L609 | L610 L611 L612 L613 L614 L615 | L616 L617 L618 L619 L620 L621 | L622 L623 L624 L625 L626 L627 | L628 L629 L630 L631 L632 L633 | L634 L635 L636 L637 L638 L639 | L640 L641 L642 L643 L644 L645 | L646 L647 L648 L649 L650 L651 | L652 L653 L654 L655 L656 L657 | L658 L659 L660 L661 L662 L663 | L664 L665 L666 L667 L668 L669 | L670 L671 L672 L673 L674 L675 | L676 L677 L678 L679 L680 L681 | L682 L683 L684 L685 L686 L687 | L688 L689 L690 L691 L692 L693 | L694 L695 L696 L697 L698 L699 | L700 L701 L702 L703 L704 L705 | L706 L707 L708 L709 L710 L711 | L712 L713 L714 L715 L716 L717 | L718 L719 L720 L721 L722 L723 | L724 L725 L726 L727 L728 L729 | L730 L731 L732 L733 L734 L735 | L736 L737 L738 L739 L740 L741 | L742 L743 L744 L745 L746 L747 | L748 L749 L750 L751 L752 L753 | L754 L755 L756 L757 L758 L759 | L760 L761 L762 L763 L764 L765 | L766 L767 L768 L769 L770 L771 | L772 L773 L774 L775 L776 L777 | L778 L779 L780 L781 L782 L783 | L784 L785 L786 L787 L788 L789 | L790 L791 L792 L793 L794 L795 | L796 L797 L798 L799 L800 L801 | L802 L803 L804 L805 L806 L807 | L808 L809 L810 L811 L812 L813 | L814 L815 L816 L817 L818 L819 | L820 L821 L822 L823 L824 L825 | L826 L827 L828 L829 L830 L831 | L832 L833 L834 L835 L836 L837 | L838 L839 L840 L841 L842 L843 | L844 L845 L846 L847 L848 L849 | L850 L851 L852 L853 L854 L855 | L856 L857 L858 L859 L860 L861 | L862 L863 L864 L865 L866 L867 | L868 L869 L870 L871 L872 L873 | L874 L875 L876 L877 L878 L879 | L880 L881 L882 L883 L884 L885 | L886 L887 L888 L889 L890 L891 | L892 L893 L894 L895 L896 L897 | L898 L899 L900 L901 L902 L903 | L904 L905 L906 L907 L908 L909 | L910 L911 L912 L913 L914 L915 | L916 L917 L918 L919 L920 L921 | L922 L923 L924 L925 L926 L927 | L928 L929 L930 L931 L932 L933 | L934 L935 L936 L937 L938 L939 | L940 L941 L942 L943 L944 L945 | L946 L947 L948 L949 L950 L951 | L952 L953 L954 L955 L956 L957 | L958 L959 L960 L961 L962 L963 | L964 L965 L966 L967 L968 L969 | L970 L971 L972 L973 L974 L975 | L976 L977 L978 L979 L980 L981 | L982 L983 L984 L985 L986 L987 | L988 L989 L990 L991 L992 L993 | L994 L995 L996 L997 L998 L999 | L1000 L1001 L1002 L1003 L1004 L1005 | L1006 L1007 L1008 L1009 L1010 L1011